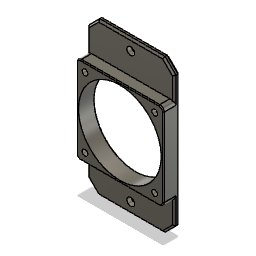
40mm-fan-mount (Autodesk Fusion 360 design; units mm, degrees)
Autodesk Fusion 360 part; units mm, degrees
sketch "Sketch1" plane through (0, 0, 0) normal (0, 0, 1) x (1, 0, 0)
  line L0 (0, 35) -> (0, -35)
  line L1 (-20, 0) -> (20, 0)
  line L2 (-15, 35) -> (15, 35)
  line L3 (20, 30) -> (20, -30)
  line L4 (15, -35) -> (-15, -35)
  line L5 (-20, -30) -> (-20, 30)
  circle A0 centre (0, 0) radius 19
  circle A1 centre (-16, 16) radius 1.3125
  circle A2 centre (16, 16) radius 1.3125
  circle A3 centre (16, -16) radius 1.3125
  circle A4 centre (-16, -16) radius 1.3125
  line L6 (-20, 20) -> (20, 20)
  line L7 (20, 20) -> (20, -20)
  line L8 (20, -20) -> (-20, -20)
  line L9 (-20, -20) -> (-20, 20)
  arc A5 (0, 16.0005) -> (0, 15.9995) centre (5, 16) ccw
  arc A6 (0, -15.9995) -> (0, -16.0005) centre (5, -16) ccw
  circle A7 centre (0, 30) radius 1.75
  circle A8 centre (0, -30) radius 1.75
  line L10 (-20, 30) -> (-15, 35)
  line L11 (15, 35) -> (20, 30)
  line L12 (-20, -30) -> (-15, -35)
  line L13 (20, -30) -> (15, -35)
  arc A9 (-20, 13) -> (-15.472, 11.028) centre (-16, 16) ccw
  arc A10 (-11.028, 15.472) -> (-13, 20) centre (-16, 16) ccw
  arc A11 (13, 20) -> (11.028, 15.472) centre (16, 16) ccw
  arc A12 (15.472, 11.028) -> (20, 13) centre (16, 16) ccw
  arc A13 (20, -13) -> (15.472, -11.028) centre (16, -16) ccw
  arc A14 (11.028, -15.472) -> (13, -20) centre (16, -16) ccw
  arc A15 (-13, -20) -> (-11.028, -15.472) centre (-16, -16) ccw
  arc A16 (-15.472, -11.028) -> (-20, -13) centre (-16, -16) ccw
  dimension "d1" = 40
  dimension "d2" = 70
  dimension "d3" = 38
  dimension "d6" = 2.625
  dimension "d7" = 16
  dimension "d8" = 16
  dimension "d10" = 32
  dimension "d13" = 40
  dimension "d14" = 5
  dimension "d15" = 3.5
  dimension "d16" = 60
  dimension "d18" = 5
  dimension "d19" = 5
  dimension "d20" = 5
  dimension "d31" = 16
  constraint vertical L0
  constraint horizontal L1
  constraint horizontal A0.centre L1.start
  constraint vertical A0.centre L0.start
  constraint symmetric L0 L1.start L1.end
  constraint symmetric L0.start L0.end L1
  constraint horizontal L2
  constraint vertical L3
  constraint horizontal L4
  constraint vertical L5
  constraint vertical L1.end L3.end
  constraint coincident L1 A0.centre
  constraint equal A1 A2
  constraint equal A1 A4
  constraint equal A1 A3
  constraint horizontal A1.centre A2.centre
  constraint vertical A1.centre A4.centre
  constraint horizontal A3.centre A4.centre
  constraint vertical A2.centre A3.centre
  constraint concentric A1 A9
  constraint concentric A4 A15
  constraint equal A9 A15
  constraint horizontal L6
  constraint vertical L7
  constraint horizontal L8
  constraint vertical L9
  constraint coincident L3 L7.end
  constraint coincident L5 L6.start
  constraint symmetric L1 L6.start L8.end
  constraint coincident L6 A10.end
  constraint coincident L8 A15.start
  constraint coincident L0 A5.end
  constraint coincident L0 A5.start
  constraint coincident L0 A6.start
  constraint coincident L0 A6.end
  constraint vertical A7.centre A8.centre
  constraint symmetric L1 A7.centre A8.centre
  constraint horizontal L5.end L3.start
  constraint horizontal L0.start L2.start
  constraint vertical L1.start L5.end
  constraint coincident L3 L13.start
  constraint perpendicular L12 L13
  constraint vertical L2.start L4.end
  constraint coincident L3.end L13.start
  constraint vertical L2.end L4.start
  constraint horizontal L5.start L3.end
  constraint horizontal L0.end L4.end
  constraint coincident A0.centre origin
  constraint concentric A2 A11
  constraint concentric A3 A13
  constraint equal A11 A13
  constraint equal A9 A13
  constraint coincident L6 A11.start
  constraint coincident L8 A14.end
  constraint vertical A0.centre A7.centre
  constraint equal A7 A8
  constraint coincident A0 A9.end
  constraint coincident A0 A10.start
  constraint concentric A9 A10
  constraint coincident L5 A9.start
  constraint coincident A0 A11.end
  constraint coincident A0 A12.start
  constraint concentric A11 A12
  constraint coincident L3 A12.end
  constraint coincident A0 A13.end
  constraint coincident A0 A14.start
  constraint concentric A13 A14
  constraint coincident L3 A13.start
  constraint coincident L5 A16.end
  constraint coincident A0 A15.end
  constraint coincident A0 A16.start
  constraint concentric A15 A16
  constraint equal A9 A10
  constraint equal A9 A12
  constraint equal A13 A14
  constraint equal A15 A16
  measures "d1" distance of L1.start L1.end
  measures "d2" distance of L0.start L0.end
  measures "d3" diameter of A0
  measures "d6" diameter of A1
  measures "d7" horizontal distance of A0.centre A1.centre
  measures "d8" vertical distance of A0.centre A1.centre
  measures "d10" distance of A1.centre A4.centre
  measures "d13" distance of L6.start L8.end
  measures "d14" radius of A9
  measures "d15" diameter of A7
  measures "d16" distance of A7.centre A8.centre
  measures "d18" horizontal distance of L5.end L2.start
  measures "d19" vertical distance of L5.end L2.start
  measures "d20" horizontal distance of L2.end L3.start
  measures "d31" horizontal distance of A0.centre A2.centre
extrude "Extrude1" add sketch "Sketch1" along normal blind 2.5 contours L0 L2 L3 L6 A5 A7 L11 | L0 L2 L5 L6 A7 L10 | L0 A0 L6 A5 | L0 A0 L6 A10 | L5 A0 L6 L9 A9 A10 | L3 A0 L6 L7 A11 A12 | L6 A5 | A0 L6 A5 | L1 L5 A0 L9 A9 | L1 L3 A0 L7 A12 | A0 L6 A5 A11 | L1 L5 A0 L9 A16 | L1 L3 A0 L7 A13 | L5 A0 L8 L9 A15 A16 | L3 A0 L7 L8 A13 A14 | L0 L4 L5 L8 A8 L12 | L0 L3 L4 L8 A6 A8 L13 | L0 A0 L8 A6 | L0 A0 L8 A15 | A0 L8 A6 | A0 L8 A6 A14 | L8 A6
extrude "Extrude2" add sketch "Sketch1" along normal blind 7.5 contours L0 A0 L6 A5 | L0 A0 L6 A10 | L5 A0 L6 L9 A9 A10 | L3 A0 L6 L7 A11 A12 | A0 L6 A5 | L1 L5 A0 L9 A9 | L1 L3 A0 L7 A12 | A0 L6 A5 A11 | L1 L5 A0 L9 A16 | L1 L3 A0 L7 A13 | L5 A0 L8 L9 A15 A16 | L3 A0 L7 L8 A13 A14 | L0 A0 L8 A6 | L0 A0 L8 A15 | A0 L8 A6 | A0 L8 A6 A14
fillet "Fillet2" radius 2 4 edges at (20, 20, 5) (20, -20, 5) (-20, 20, 5) (-20, -20, 5)
chamfer "Chamfer1" distance 0.4 angle 45 8 edges at (0, 20, 7.5) (-19.4142, 19.4142, 7.5) (-20, 0, 7.5) (-19.4142, -19.4142, 7.5) (0, -20, 7.5) (19.4142, -19.4142, 7.5) (20, 0, 7.5) (19.4142, 19.4142, 7.5)
chamfer "Chamfer2" distance 0.8 angle 45 20 edges at (20, 25, 2.5) (20, -25, 2.5) (20, -25, 2.5) (17.5, 32.5, 2.5) (0, 35, 2.5) (-17.5, 32.5, 2.5) (-20, 25, 2.5) (-20, 25, 2.5) (-20, -25, 2.5) (-17.5, -32.5, 2.5) (0, -35, 2.5) (17.5, -32.5, 2.5) (20, 0, 0) (17.5, 32.5, 0) (0, 35, 0) (-17.5, 32.5, 0) (-20, 0, 0) (-17.5, -32.5, 0) (0, -35, 0) (17.5, -32.5, 0)
chamfer "Chamfer3" distance 0.4 angle 45 7 edges at (14.7763, 16.4746, 0) (-1.6316, 30.6328, 0) (-17.2237, 16.4746, 0) (-17.7142, 6.8707, 0) (-17.2237, -15.5254, 0) (-1.6316, -29.3672, 0) (14.7763, -15.5254, 0)
